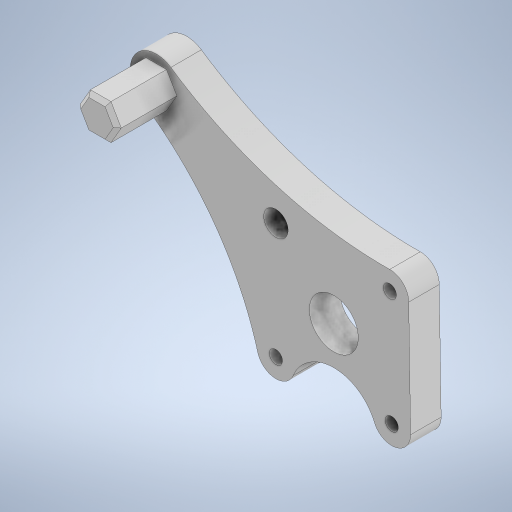
# Autodesk Inventor part: ArmGearMount
Saved by Autodesk Inventor 2023 (Build 270158030, 158C)
## iProperties
Created: 2024-10-17
Part Number: ArmGearMount
Material: Generic
Document SubType Name: Modeling
Designer: lvrectanus0
Density: 1 g/cm^3
Appearance: Default
Author: lvrectanus0
Autodesk Inventor part; units mm, degrees
ref_plane "YZ Plane" through (0, 0, 0) normal (1, 0, 0) x (0, 1, 0)
ref_plane "XZ Plane" through (0, 0, 0) normal (0, 1, 0) x (-1, 0, 0)
ref_plane "XY Plane" through (0, 0, 0) normal (0, 0, 1) x (1, 0, 0)
sketch "Sketch1" plane through (0, 0, 0) normal (0, 0, 1) x (1, 0, 0)
  circle A0 centre (9.5, 9.5) radius 2.5 projected
  circle A1 centre (40, 40) radius 2.5 projected
  circle A2 centre (40.5, 9.5) radius 2.5 projected
  circle A3 centre (9.5, 40.5) radius 2.5 projected
  line L0 (47.46, 3) -> (27.54, 3) projected
  line L1 (47.46, 3) -> (47.46, 12.7) projected
  line L2 (47.46, 12.7) -> (50, 12.7) projected
  line L3 (50, 12.7) -> (50, 40) projected
  arc A4 (50, 40) -> (40, 50) centre (40, 40) ccw projected
  line L4 (10, 50) -> (40, 50) projected
  arc A5 (10, 50) -> (0, 40) centre (10, 40) ccw projected
  line L5 (0, 12.7) -> (0, 40) projected
  line L6 (0, 12.7) -> (2.54, 12.7) projected
  line L7 (2.54, 12.7) -> (2.54, 3) projected
  line L8 (22.46, 3) -> (2.54, 3) projected
  line L9 (22.46, 3) -> (22.46, 12.7) projected
  line L10 (22.46, 12.7) -> (27.54, 12.7) projected
  line L11 (27.54, 12.7) -> (27.54, 3) projected
  circle A6 centre (25, 25) radius 4 projected
  line L12 (25, 25) -> (-22.519, 56.75) construction
  line L13 (-22.519, 56.75) -> (25, 56.75) construction
  line L14 (25, 56.75) -> (25, 25) construction
  line L15 (-28.0183, 56.75) -> (-25.2687, 61.5125)
  line L16 (-25.2687, 61.5125) -> (-19.7694, 61.5125)
  line L17 (-19.7694, 61.5125) -> (-17.0198, 56.75)
  line L18 (-17.0198, 56.75) -> (-19.7694, 51.9875)
  line L19 (-19.7694, 51.9875) -> (-25.2687, 51.9875)
  line L20 (-25.2687, 51.9875) -> (-28.0183, 56.75)
  line L21 (-19.7694, 61.5125) -> (-25.2687, 51.9875) construction
  circle A7 centre (-22.519, 56.75) radius 6.985
  circle A8 centre (40, 40) radius 5.04
  circle A9 centre (40.5, 9.5) radius 5.04
  circle A10 centre (9.5, 9.5) radius 5.04
  arc A11 (35.8521, 7.5509) -> (14.1479, 7.5509) centre (25, 3) ccw
  arc A12 (4.6471, 8.1396) -> (-26.3996, 50.9421) centre (-68.7442, -12.4335) ccw
  arc A13 (-18.6385, 62.5579) -> (39.9595, 45.0398) centre (39.1237, 149.0084) ccw
  circle A14 centre (25, 25) radius 6.54
  line L22 (-26.3996, 50.9421) -> (-15.682, 43.7811) construction
  line L23 (-18.6385, 62.5579) -> (-6.4516, 54.4152) construction
  line L24 (45.54, 9.5) -> (45.04, 40)
  circle A15 centre (40, 40) radius 1.75 projected
  circle A16 centre (40.5, 9.5) radius 1.75 projected
  circle A17 centre (9.5, 9.5) radius 1.75 projected
  circle A18 centre (9.5, 40.5) radius 3.2571
  point P0 (0, 0)
  dimension "d0" = 57.15
  dimension "d1" = 31.75
  dimension "d3" = 120
  dimension "d4" = 120
  dimension "d5" = 9.525
  dimension "d6" = 13.97
  dimension "d7" = 2.54
  dimension "d8" = 2.54
  dimension "d9" = 2.54
  dimension "d11" = 2.54
  constraints: 26 end point, 14 point on circle, 9 centre point, 9 tangent, 5 equal length, 4 parallel, 2 coincident, 2 horizontal, 1 horizontal alignment, 1 midpoint, 1 point on line, 1 vertical
  measures "d0" distance of L12.start L12.end
  measures "d1" distance of L13.end L12.start
  measures "d3" angle of L20 L15
  measures "d4" angle of L16 L17
  measures "d5" distance between parallel lines of L19 L16
  measures "d6" diameter of A7
  measures "d7" radial gap between concentric circles of A1 A8
  measures "d8" radial gap between concentric circles of A2 A9
  measures "d9" radial gap between concentric circles of A0 A10
  measures "d11" radial gap between concentric circles of A6 A14
extrude "Extrusion1" add sketch "Sketch1" along normal blind 8.175 contours A0 | A1 | A2 | A9 | A13 A8 L24 A9 A11 A10 A12 L5 A5 | A5 L5 A12 A7 A13 | A7 | A8 | A10 | L15 L16 L17 L18 L19 L20
sketch "Sketch2" plane through (0, 0, 8.175) normal (0, 0, 1) x (1, 0, 0)
  line L0 (-25.2687, 51.9875) -> (-28.0183, 56.75) projected
  line L1 (-28.0183, 56.75) -> (-25.2687, 61.5125) projected
  line L2 (-25.2687, 61.5125) -> (-19.7694, 61.5125) projected
  line L3 (-19.7694, 61.5125) -> (-17.0198, 56.75) projected
  line L4 (-17.0198, 56.75) -> (-19.7694, 51.9875) projected
  line L5 (-19.7694, 51.9875) -> (-25.2687, 51.9875) projected
  point P0 (0, 0)
extrude "Extrusion2" add sketch "Sketch2" along normal blind 15.875
chamfer "Chamfer1" distance 1 angle 45 6 edges at (-22.519, 61.5125, 24.05) (-26.6435, 59.1312, 24.05) (-26.6435, 54.3687, 24.05) (-22.519, 51.9875, 24.05) (-18.3946, 59.1312, 24.05) (-18.3946, 54.3687, 24.05)
body "Solid1"
